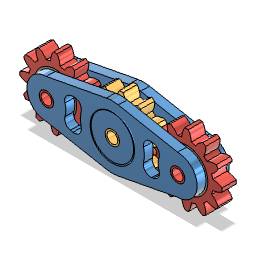
spur_gear_spinner (Autodesk Fusion 360 design; units mm, degrees)
Autodesk Fusion 360 part; units mm, degrees
sketch "Sketch1" plane through (0, 0, 0) normal (0, 0, 1) x (1, 0, 0)
  circle A0 centre (100, 50) radius 4
  circle A1 centre (174, 50) radius 4
  circle A2 centre (137.1972, 50) radius 12
  line L0 (100, 61) -> (133.8504, 67.3702)
  line L1 (140.5427, 67.3637) -> (174, 61)
  line L2 (100, 39) -> (133.8504, 32.6298)
  line L3 (140.5427, 32.6363) -> (174, 39)
  line L4 (113.559, 58.4638) -> (114.9878, 58.7327)
  line L5 (113.559, 41.5362) -> (114.9878, 41.2673)
  line L6 (159.425, 58.6826) -> (160.4563, 58.4864)
  line L7 (159.425, 41.3174) -> (160.4563, 41.5136)
  arc A3 (140.5427, 67.3637) -> (133.8504, 67.3702) centre (137.1794, 49.6807) ccw
  arc A4 (133.8504, 32.6298) -> (140.5427, 32.6363) centre (137.1794, 50.3193) ccw
  arc A5 (113.559, 58.4638) -> (110.4857, 53.3241) centre (114.2987, 54.5328) ccw
  arc A6 (119.6312, 53.9287) -> (114.9878, 58.7327) centre (115.7276, 54.8017) ccw
  arc A7 (100, 61) -> (100, 39) centre (100, 50) ccw
  arc A8 (110.4857, 46.6759) -> (110.4857, 53.3241) centre (100, 50) ccw
  arc A9 (119.6312, 53.9287) -> (119.6312, 46.0713) centre (137.1972, 50) ccw
  arc A10 (154.7721, 46.1112) -> (154.7721, 53.8888) centre (137.1972, 50) ccw
  arc A11 (163.5199, 53.3417) -> (163.5199, 46.6583) centre (174, 50) ccw
  arc A12 (174, 39) -> (174, 61) centre (174, 50) ccw
  arc A13 (110.4857, 46.6759) -> (113.559, 41.5362) centre (114.2987, 45.4672) ccw
  arc A14 (114.9878, 41.2673) -> (119.6312, 46.0713) centre (115.7276, 45.1983) ccw
  arc A15 (159.425, 58.6826) -> (154.7721, 53.8888) centre (158.6776, 54.753) ccw
  arc A16 (163.5199, 53.3417) -> (160.4563, 58.4864) centre (159.7089, 54.5569) ccw
  arc A17 (154.7721, 46.1112) -> (159.425, 41.3174) centre (158.6776, 45.247) ccw
  arc A18 (160.4563, 41.5136) -> (163.5199, 46.6583) centre (159.7089, 45.4431) ccw
  line L8 (300, 39) -> (266.1496, 32.6298)
  circle A19 centre (300, 50) radius 4
  arc A20 (266.1496, 67.3702) -> (259.4573, 67.3637) centre (262.8206, 49.6807) ccw
  arc A21 (240.575, 41.3174) -> (245.2279, 46.1112) centre (241.3224, 45.247) ccw
  line L9 (240.575, 58.6826) -> (239.5437, 58.4864)
  line L10 (259.4573, 32.6363) -> (226, 39)
  line L11 (300, 61) -> (266.1496, 67.3702)
  arc A22 (236.4801, 46.6583) -> (239.5437, 41.5136) centre (240.2911, 45.4431) ccw
  arc A23 (280.3688, 46.0713) -> (285.0122, 41.2673) centre (284.2724, 45.1983) ccw
  arc A24 (245.2279, 53.8888) -> (245.2279, 46.1112) centre (262.8028, 50) ccw
  arc A25 (286.441, 41.5362) -> (289.5143, 46.6759) centre (285.7013, 45.4672) ccw
  line L12 (286.441, 41.5362) -> (285.0122, 41.2673)
  arc A26 (239.5437, 58.4864) -> (236.4801, 53.3417) centre (240.2911, 54.5569) ccw
  arc A27 (289.5143, 53.3241) -> (289.5143, 46.6759) centre (300, 50) ccw
  arc A28 (245.2279, 53.8888) -> (240.575, 58.6826) centre (241.3224, 54.753) ccw
  arc A29 (285.0122, 58.7327) -> (280.3688, 53.9287) centre (284.2724, 54.8017) ccw
  line L13 (240.575, 41.3174) -> (239.5437, 41.5136)
  arc A30 (236.4801, 46.6583) -> (236.4801, 53.3417) centre (226, 50) ccw
  circle A31 centre (262.8028, 50) radius 12
  arc A32 (226, 61) -> (226, 39) centre (226, 50) ccw
  arc A33 (289.5143, 53.3241) -> (286.441, 58.4638) centre (285.7013, 54.5328) ccw
  arc A34 (259.4573, 32.6363) -> (266.1496, 32.6298) centre (262.8206, 50.3193) ccw
  arc A35 (300, 39) -> (300, 61) centre (300, 50) ccw
  circle A36 centre (226, 50) radius 4
  line L14 (259.4573, 67.3637) -> (226, 61)
  line L15 (286.441, 58.4638) -> (285.0122, 58.7327)
  arc A37 (280.3688, 46.0713) -> (280.3688, 53.9287) centre (262.8028, 50) ccw
  dimension "d1" = 22
  dimension "d2" = 8
  dimension "d3" = 22
  dimension "d4" = 8
  dimension "d5" = 74
  dimension "d6" = 36
  dimension "d7" = 24
  dimension "d8" = 5
  dimension "d9" = 5
  dimension "d11" = 5
  dimension "d12" = 5
  dimension "d13" = 18
  dimension "d14" = 18
  dimension "d15" = 4
  dimension "d16" = 4
  dimension "d17" = 4
  dimension "d18" = 4
  dimension "d19" = 4
  dimension "d20" = 4
  dimension "d21" = 4
  dimension "d22" = 4
  constraint concentric A0 A7
  constraint concentric A1 A11
  constraint concentric A2 A9
  constraint coincident L3.end A11
  constraint parallel L0 L4
  constraint parallel L2 L5
  constraint parallel L1 L6
  constraint parallel L3 L7
  constraint tangent L0 A3
  constraint tangent L1 A3
  constraint tangent L2 A4
  constraint tangent L3 A4
  constraint tangent A5 A7
  constraint tangent L4 A5
  constraint tangent L4 A6
  constraint tangent A6 A9
  constraint concentric A7 A8
  constraint concentric A9 A10
  constraint concentric A11 A12
  constraint tangent A8 A13
  constraint tangent L5 A13
  constraint tangent L5 A14
  constraint tangent A9 A14
  constraint tangent A10 A15
  constraint tangent L6 A15
  constraint tangent L6 A16
  constraint tangent A11 A16
  constraint tangent A10 A17
  constraint tangent L7 A17
  constraint tangent L7 A18
  constraint tangent A11 A18
  measures "d1" diameter of A7
  measures "d2" diameter of A0
  measures "d3" diameter of A11
  measures "d4" diameter of A1
  measures "d5" distance of A0.centre A1.centre
  measures "d6" diameter of A9
  measures "d7" diameter of A2
  measures "d8" distance of L0 L4
  measures "d9" distance of L2 L5
  measures "d11" distance of L1 L6
  measures "d12" distance of L3 L7
  measures "d13" radius of A3
  measures "d14" radius of A4
  measures "d15" radius of A5
  measures "d16" radius of A6
  measures "d17" radius of A13
  measures "d18" radius of A14
  measures "d19" radius of A15
  measures "d20" radius of A16
  measures "d21" radius of A17
  measures "d22" radius of A18
extrude "Extrude1" add sketch "Sketch1" along normal blind 5 contours L0 L1 L2 L3 A3 A4 A7 A12 makes body 1 in component "Top plate"
extrude "Extrude1'" add sketch "Sketch1" along normal blind 5 separate body contours L8 A20 L10 L11 A32 A34 A35 L14 makes body 2 in component "Bottom plate"
sketch "Sketch2" plane through (0, 0, 0) normal (0, 0, 1) x (1, 0, 0)
  circle A0 centre (98.0968, 130.2968) radius 12
  line L0 (97.0968, 150.2968) -> (99.0968, 150.2968)
  arc A1 (97.0968, 150.2968) -> (95.4218, 145.0564) centre (105.4171, 144.7495) ccw
  arc A2 (100.7718, 145.0564) -> (99.0968, 150.2968) centre (90.7765, 144.7495) ccw
  arc A3 (93.0336, 144.4165) -> (88.9628, 148.1173) centre (84.5309, 139.1531) ccw
  line L1 (87.2307, 147.1173) -> (88.9628, 148.1173)
  arc A4 (87.2307, 147.1173) -> (88.4004, 141.7415) centre (97.21, 146.4734) ccw
  arc A5 (86.6521, 139.9932) -> (81.2763, 141.1629) centre (81.9202, 131.1836) ccw
  line L2 (80.2763, 139.4308) -> (81.2763, 141.1629)
  arc A6 (80.2763, 139.4308) -> (83.9771, 135.36) centre (89.2405, 143.8627) ccw
  arc A7 (83.3372, 132.9718) -> (78.0968, 131.2968) centre (83.6441, 122.9765) ccw
  line L3 (78.0968, 129.2968) -> (78.0968, 131.2968)
  arc A8 (78.0968, 129.2968) -> (83.3372, 127.6218) centre (83.6441, 137.6171) ccw
  arc A9 (83.9771, 125.2337) -> (80.2763, 121.1629) centre (89.2405, 116.7309) ccw
  line L4 (81.2763, 119.4308) -> (80.2763, 121.1629)
  arc A10 (81.2763, 119.4308) -> (86.6521, 120.6004) centre (81.9202, 129.4101) ccw
  arc A11 (88.4004, 118.8522) -> (87.2307, 113.4763) centre (97.21, 114.1203) ccw
  line L5 (88.9628, 112.4763) -> (87.2307, 113.4763)
  arc A12 (88.9628, 112.4763) -> (93.0336, 116.1772) centre (84.5309, 121.4406) ccw
  arc A13 (95.4218, 115.5373) -> (97.0968, 110.2968) centre (105.4171, 115.8442) ccw
  line L6 (99.0968, 110.2968) -> (97.0968, 110.2968)
  arc A14 (99.0968, 110.2968) -> (100.7718, 115.5373) centre (90.7765, 115.8442) ccw
  arc A15 (103.1599, 116.1772) -> (107.2307, 112.4763) centre (111.6627, 121.4406) ccw
  line L7 (108.9628, 113.4763) -> (107.2307, 112.4763)
  arc A16 (108.9628, 113.4763) -> (107.7932, 118.8522) centre (98.9835, 114.1203) ccw
  arc A17 (109.5414, 120.6004) -> (114.9173, 119.4308) centre (114.2733, 129.4101) ccw
  line L8 (115.9173, 121.1629) -> (114.9173, 119.4308)
  arc A18 (115.9173, 121.1629) -> (112.2164, 125.2337) centre (106.953, 116.7309) ccw
  arc A19 (112.8563, 127.6218) -> (118.0968, 129.2968) centre (112.5494, 137.6171) ccw
  line L9 (118.0968, 131.2968) -> (118.0968, 129.2968)
  arc A20 (118.0968, 131.2968) -> (112.8563, 132.9718) centre (112.5494, 122.9765) ccw
  arc A21 (112.2164, 135.36) -> (115.9173, 139.4308) centre (106.953, 143.8627) ccw
  line L10 (114.9173, 141.1629) -> (115.9173, 139.4308)
  arc A22 (114.9173, 141.1629) -> (109.5414, 139.9932) centre (114.2733, 131.1836) ccw
  arc A23 (107.7932, 141.7415) -> (108.9628, 147.1173) centre (98.9835, 146.4734) ccw
  line L11 (107.2307, 148.1173) -> (108.9628, 147.1173)
  arc A24 (107.2307, 148.1173) -> (103.1599, 144.4165) centre (111.6627, 139.1531) ccw
  arc A25 (103.1599, 144.4165) -> (100.7718, 145.0564) centre (98.0968, 130.2968) ccw
  arc A26 (109.5414, 139.9932) -> (107.7932, 141.7415) centre (98.0968, 130.2968) ccw
  arc A27 (112.8563, 132.9718) -> (112.2164, 135.36) centre (98.0968, 130.2968) ccw
  arc A28 (112.2164, 125.2337) -> (112.8563, 127.6218) centre (98.0968, 130.2968) ccw
  arc A29 (107.7932, 118.8522) -> (109.5414, 120.6004) centre (98.0968, 130.2968) ccw
  arc A30 (100.7718, 115.5373) -> (103.1599, 116.1772) centre (98.0968, 130.2968) ccw
  arc A31 (93.0336, 116.1772) -> (95.4218, 115.5373) centre (98.0968, 130.2968) ccw
  arc A32 (86.6521, 120.6004) -> (88.4004, 118.8522) centre (98.0968, 130.2968) ccw
  arc A33 (83.3372, 127.6218) -> (83.9771, 125.2337) centre (98.0968, 130.2968) ccw
  arc A34 (83.9771, 135.36) -> (83.3372, 132.9718) centre (98.0968, 130.2968) ccw
  arc A35 (95.4218, 145.0564) -> (93.0336, 144.4165) centre (98.0968, 130.2968) ccw
  arc A36 (88.4004, 141.7415) -> (86.6521, 139.9932) centre (98.0968, 130.2968) ccw
  arc A37 (151.0372, 147.1173) -> (152.2068, 141.7415) centre (161.0165, 146.4734) ccw
  circle A38 centre (161.9032, 130.2968) radius 12
  arc A39 (164.5782, 145.0564) -> (162.9032, 150.2968) centre (154.5829, 144.7495) ccw
  arc A40 (173.3479, 139.9932) -> (171.5996, 141.7415) centre (161.9032, 130.2968) ccw
  arc A41 (176.0229, 135.36) -> (179.7237, 139.4308) centre (170.7595, 143.8627) ccw
  arc A42 (164.5782, 115.5373) -> (166.9664, 116.1772) centre (161.9032, 130.2968) ccw
  line L12 (172.7693, 147.1173) -> (171.0372, 148.1173)
  arc A43 (176.0229, 125.2337) -> (176.6628, 127.6218) centre (161.9032, 130.2968) ccw
  arc A44 (172.7693, 113.4763) -> (171.5996, 118.8522) centre (162.79, 114.1203) ccw
  arc A45 (171.5996, 118.8522) -> (173.3479, 120.6004) centre (161.9032, 130.2968) ccw
  line L13 (179.7237, 139.4308) -> (178.7237, 141.1629)
  arc A46 (171.5996, 141.7415) -> (172.7693, 147.1173) centre (162.79, 146.4734) ccw
  line L14 (181.9032, 129.2968) -> (181.9032, 131.2968)
  arc A47 (179.7237, 121.1629) -> (176.0229, 125.2337) centre (170.7595, 116.7309) ccw
  arc A48 (176.6628, 127.6218) -> (181.9032, 129.2968) centre (176.3559, 137.6171) ccw
  line L15 (178.7237, 119.4308) -> (179.7237, 121.1629)
  line L16 (144.0827, 121.1629) -> (145.0827, 119.4308)
  arc A49 (144.0827, 139.4308) -> (147.7836, 135.36) centre (153.047, 143.8627) ccw
  arc A50 (147.1437, 127.6218) -> (147.7836, 125.2337) centre (161.9032, 130.2968) ccw
  arc A51 (159.2282, 115.5373) -> (160.9032, 110.2968) centre (169.2235, 115.8442) ccw
  arc A52 (147.7836, 125.2337) -> (144.0827, 121.1629) centre (153.047, 116.7309) ccw
  line L17 (145.0827, 141.1629) -> (144.0827, 139.4308)
  arc A53 (147.7836, 135.36) -> (147.1437, 132.9718) centre (161.9032, 130.2968) ccw
  arc A54 (160.9032, 150.2968) -> (159.2282, 145.0564) centre (169.2235, 144.7495) ccw
  arc A55 (145.0827, 119.4308) -> (150.4586, 120.6004) centre (145.7267, 129.4101) ccw
  arc A56 (152.2068, 118.8522) -> (151.0372, 113.4763) centre (161.0165, 114.1203) ccw
  arc A57 (152.7693, 112.4763) -> (156.8401, 116.1772) centre (148.3373, 121.4406) ccw
  arc A58 (141.9032, 129.2968) -> (147.1437, 127.6218) centre (147.4506, 137.6171) ccw
  line L18 (141.9032, 131.2968) -> (141.9032, 129.2968)
  arc A59 (159.2282, 145.0564) -> (156.8401, 144.4165) centre (161.9032, 130.2968) ccw
  arc A60 (150.4586, 139.9932) -> (145.0827, 141.1629) centre (145.7267, 131.1836) ccw
  arc A61 (166.9664, 116.1772) -> (171.0372, 112.4763) centre (175.4691, 121.4406) ccw
  arc A62 (173.3479, 120.6004) -> (178.7237, 119.4308) centre (178.0798, 129.4101) ccw
  arc A63 (166.9664, 144.4165) -> (164.5782, 145.0564) centre (161.9032, 130.2968) ccw
  arc A64 (171.0372, 148.1173) -> (166.9664, 144.4165) centre (175.4691, 139.1531) ccw
  arc A65 (181.9032, 131.2968) -> (176.6628, 132.9718) centre (176.3559, 122.9765) ccw
  line L19 (152.7693, 148.1173) -> (151.0372, 147.1173)
  arc A66 (162.9032, 110.2968) -> (164.5782, 115.5373) centre (154.5829, 115.8442) ccw
  line L20 (171.0372, 112.4763) -> (172.7693, 113.4763)
  arc A67 (178.7237, 141.1629) -> (173.3479, 139.9932) centre (178.0798, 131.1836) ccw
  arc A68 (156.8401, 116.1772) -> (159.2282, 115.5373) centre (161.9032, 130.2968) ccw
  arc A69 (156.8401, 144.4165) -> (152.7693, 148.1173) centre (148.3373, 139.1531) ccw
  arc A70 (176.6628, 132.9718) -> (176.0229, 135.36) centre (161.9032, 130.2968) ccw
  line L21 (151.0372, 113.4763) -> (152.7693, 112.4763)
  arc A71 (147.1437, 132.9718) -> (141.9032, 131.2968) centre (147.4506, 122.9765) ccw
  arc A72 (152.2068, 141.7415) -> (150.4586, 139.9932) centre (161.9032, 130.2968) ccw
  arc A73 (150.4586, 120.6004) -> (152.2068, 118.8522) centre (161.9032, 130.2968) ccw
  line L22 (162.9032, 150.2968) -> (160.9032, 150.2968)
  line L23 (160.9032, 110.2968) -> (162.9032, 110.2968)
  dimension "d27" = 30
  dimension "d28" = 24
  dimension "d29" = 20
  dimension "d36" = 10
  dimension "d38" = 360
  constraint concentric A0 A35
  constraint horizontal L0
  constraint concentric A25 A35
  constraint concentric A26 A35
  constraint concentric A27 A35
  constraint concentric A28 A35
  constraint concentric A29 A35
  constraint concentric A30 A35
  constraint concentric A31 A35
  constraint concentric A32 A35
  constraint concentric A33 A35
  constraint concentric A34 A35
  constraint concentric A35 A36
  measures "d27" diameter of A35
  measures "d28" diameter of A0
  measures "d29" distance of A0.centre L0
  measures "d36" radius of A1
extrude "Extrude1''" add sketch "Sketch2" along normal blind 8 separate body contours L0 A1 A2 A3 L1 A4 A5 L2 A6 A7 L3 A8 A9 L4 A10 A11 L5 A12 A13 L6 A14 A15 L7 A16 A17 L8 A18 A19 L9 A20 A21 L10 A22 A23 L11 A24 A25 A26 A27 A28 A29 A30 A31 A32 A33 A34 A35 A36 makes body 3 in component "Spur Gear1/3"
extrude "Extrude1'''" add sketch "Sketch2" along normal blind 8 separate body contours A37 A39 A40 A41 A42 L12 A43 A44 A45 L13 A46 L14 A47 A48 L15 L16 A49 A50 A51 A52 L17 A53 A54 A55 A56 A57 A58 L18 A59 A60 A61 A62 A63 A64 A65 L19 A66 L20 A67 A68 A69 A70 L21 A71 A72 A73 L22 L23 makes body 4 in component "Spu Gear 2/3"
sketch "Sketch3" plane through (0, 0, 0) normal (0, 0, 1) x (1, 0, 0)
  circle A0 centre (243.1041, 130.2402) radius 4
  line L0 (242.1041, 150.2402) -> (244.1041, 150.2402)
  arc A1 (245.7791, 144.9998) -> (244.1041, 150.2402) centre (235.7838, 144.6929) ccw
  arc A2 (242.1041, 150.2402) -> (240.4291, 144.9998) centre (250.4244, 144.6929) ccw
  arc A3 (238.041, 144.3599) -> (233.9702, 148.0607) centre (229.5382, 139.0965) ccw
  arc A4 (232.2381, 147.0607) -> (233.4077, 141.6849) centre (242.2173, 146.4167) ccw
  line L1 (232.2381, 147.0607) -> (233.9702, 148.0607)
  arc A5 (231.6595, 139.9366) -> (226.2836, 141.1062) centre (226.9276, 131.127) ccw
  arc A6 (225.2836, 139.3742) -> (228.9845, 135.3034) centre (234.2479, 143.8061) ccw
  line L2 (225.2836, 139.3742) -> (226.2836, 141.1062)
  arc A7 (228.3446, 132.9152) -> (223.1041, 131.2402) centre (228.6514, 122.9199) ccw
  arc A8 (223.1041, 129.2402) -> (228.3446, 127.5652) centre (228.6514, 137.5605) ccw
  line L3 (223.1041, 129.2402) -> (223.1041, 131.2402)
  arc A9 (228.9845, 125.1771) -> (225.2836, 121.1062) centre (234.2479, 116.6743) ccw
  arc A10 (226.2836, 119.3742) -> (231.6595, 120.5438) centre (226.9276, 129.3534) ccw
  line L4 (226.2836, 119.3742) -> (225.2836, 121.1062)
  arc A11 (233.4077, 118.7956) -> (232.2381, 113.4197) centre (242.2173, 114.0637) ccw
  arc A12 (233.9702, 112.4197) -> (238.041, 116.1206) centre (229.5382, 121.384) ccw
  line L5 (233.9702, 112.4197) -> (232.2381, 113.4197)
  arc A13 (240.4291, 115.4807) -> (242.1041, 110.2402) centre (250.4244, 115.7875) ccw
  arc A14 (244.1041, 110.2402) -> (245.7791, 115.4807) centre (235.7838, 115.7875) ccw
  line L6 (244.1041, 110.2402) -> (242.1041, 110.2402)
  arc A15 (248.1673, 116.1206) -> (252.2381, 112.4197) centre (256.67, 121.384) ccw
  arc A16 (253.9702, 113.4197) -> (252.8005, 118.7956) centre (243.9909, 114.0637) ccw
  line L7 (253.9702, 113.4197) -> (252.2381, 112.4197)
  arc A17 (254.5488, 120.5438) -> (259.9246, 119.3742) centre (259.2807, 129.3534) ccw
  arc A18 (260.9246, 121.1062) -> (257.2238, 125.1771) centre (251.9604, 116.6743) ccw
  line L8 (260.9246, 121.1062) -> (259.9246, 119.3742)
  arc A19 (257.8637, 127.5652) -> (263.1041, 129.2402) centre (257.5568, 137.5605) ccw
  arc A20 (263.1041, 131.2402) -> (257.8637, 132.9152) centre (257.5568, 122.9199) ccw
  line L9 (263.1041, 131.2402) -> (263.1041, 129.2402)
  arc A21 (257.2238, 135.3034) -> (260.9246, 139.3742) centre (251.9604, 143.8061) ccw
  arc A22 (259.9246, 141.1062) -> (254.5488, 139.9366) centre (259.2807, 131.127) ccw
  line L10 (259.9246, 141.1062) -> (260.9246, 139.3742)
  arc A23 (252.8005, 141.6849) -> (253.9702, 147.0607) centre (243.9909, 146.4167) ccw
  arc A24 (252.2381, 148.0607) -> (248.1673, 144.3599) centre (256.67, 139.0965) ccw
  line L11 (252.2381, 148.0607) -> (253.9702, 147.0607)
  arc A25 (248.1673, 144.3599) -> (245.7791, 144.9998) centre (243.1041, 130.2402) ccw
  arc A26 (254.5488, 139.9366) -> (252.8005, 141.6849) centre (243.1041, 130.2402) ccw
  arc A27 (257.8637, 132.9152) -> (257.2238, 135.3034) centre (243.1041, 130.2402) ccw
  arc A28 (257.2238, 125.1771) -> (257.8637, 127.5652) centre (243.1041, 130.2402) ccw
  arc A29 (252.8005, 118.7956) -> (254.5488, 120.5438) centre (243.1041, 130.2402) ccw
  arc A30 (245.7791, 115.4807) -> (248.1673, 116.1206) centre (243.1041, 130.2402) ccw
  arc A31 (238.041, 116.1206) -> (240.4291, 115.4807) centre (243.1041, 130.2402) ccw
  arc A32 (231.6595, 120.5438) -> (233.4077, 118.7956) centre (243.1041, 130.2402) ccw
  arc A33 (228.3446, 127.5652) -> (228.9845, 125.1771) centre (243.1041, 130.2402) ccw
  arc A34 (228.9845, 135.3034) -> (228.3446, 132.9152) centre (243.1041, 130.2402) ccw
  arc A35 (240.4291, 144.9998) -> (238.041, 144.3599) centre (243.1041, 130.2402) ccw
  arc A36 (233.4077, 141.6849) -> (231.6595, 139.9366) centre (243.1041, 130.2402) ccw
  dimension "d43" = 30
  dimension "d44" = 8
  dimension "d45" = 20
  dimension "d51" = 10
  dimension "d53" = 360
  constraint concentric A0 A35
  constraint horizontal L0
  constraint concentric A25 A35
  constraint concentric A26 A35
  constraint concentric A27 A35
  constraint concentric A28 A35
  constraint concentric A29 A35
  constraint concentric A30 A35
  constraint concentric A31 A35
  constraint concentric A32 A35
  constraint concentric A33 A35
  constraint concentric A34 A35
  constraint concentric A35 A36
  measures "d43" diameter of A35
  measures "d44" diameter of A0
  measures "d45" distance of A0.centre L0
  measures "d51" radius of A1
extrude "Extrude1''''" add sketch "Sketch3" along normal blind 8 separate body makes body 5 in component "Spur Gear3/3"
sketch "Sketch4" plane through (0, 0, 0) normal (0, 0, 1) x (1, 0, 0)
  circle A0 centre (100, 200) radius 13
  circle A1 centre (100, 200) radius 4
  circle A2 centre (150, 200) radius 4
  circle A3 centre (150, 200) radius 13
  dimension "d56" = 26
  dimension "d57" = 8
  constraint concentric A0 A1
  measures "d56" diameter of A0
  measures "d57" diameter of A1
extrude "Extrude1'''''" add sketch "Sketch4" along normal blind 5 separate body contours A0 makes body 6 in component "major Base"
fillet "Fillet1" radius 0.5 1 edges at (87.8797, 195.299, 5) on bodies 6 in component "major Base"
fillet "Fillet2" radius 0.5 1 edges at (87.8797, 195.299, 0) on bodies 6 in component "major Base"
extrude "Extrude1''''''" add sketch "Sketch4" along normal blind 5 separate body contours A3 makes body 7 in component "pillor cap"
fillet "Fillet1'" radius 0.5 1 edges at (137.8797, 195.299, 5) on bodies 7 in component "pillor cap"
fillet "Fillet2'" radius 0.5 1 edges at (137.8797, 195.299, 0) on bodies 7 in component "pillor cap"
sketch "Sketch5" plane through (0, 0, 0) normal (0, 0, 1) x (1, 0, 0)
  circle A0 centre (200, 200) radius 4
  circle A1 centre (200, 200) radius 3
  circle A2 centre (220, 200) radius 3
  circle A3 centre (220, 200) radius 4
  circle A4 centre (240, 200) radius 3
  circle A5 centre (240, 200) radius 4
  circle A6 centre (100, 260) radius 12
  circle A7 centre (100, 260) radius 4
  circle A8 centre (150, 260) radius 4
  circle A9 centre (150, 260) radius 12
  dimension "d70" = 8
  dimension "d71" = 6
  dimension "d72" = 24
  dimension "d73" = 8
  constraint concentric A0 A1
  constraint concentric A6 A7
  measures "d70" diameter of A0
  measures "d71" diameter of A1
  measures "d72" diameter of A6
  measures "d73" diameter of A7
extrude "Extrude1'''''''" add sketch "Sketch5" along normal blind 18 separate body contours A0 makes body 8 in component "major Pillar"
extrude "Extrude1''''''''" add sketch "Sketch5" along normal blind 18 separate body contours A3 makes body 9 in component "minor pillar 1/2"
extrude "Extrude1'''''''''" add sketch "Sketch5" along normal blind 18 separate body contours A5 makes body 10 in component "minor pillar 2/2"
extrude "Extrude1''''''''''" add sketch "Sketch5" along normal blind 8 separate body contours A6 makes body 11 in component "Component"
extrude "Extrude1'''''''''''" add sketch "Sketch5" along normal blind 8 separate body contours A9 makes body 12 in component "Component'"
component "Top plate" placed x (1, 0, 0) y (0, 1, 0) z (0, 0, 1) at (0, 0, 0)
component "Bottom plate" placed x (1, 0, 0) y (0, 1, 0) z (0, 0, 1) at (-126, 0, -13)
component "Spur Gear1/3" placed x (1, 0, 0) y (0, 1, 0) z (0, 0, 1) at (1.9032, -80.2968, -8)
component "Spu Gear 2/3" placed x (1, 0, 0) y (0, 1, 0) z (0, 0, 1) at (12.0968, -80.2968, -8)
component "Spur Gear3/3" placed x (1, 0, 0) y (0, 1, 0) z (0, 0, 1) at (-105.9248, -80.5595, -8)
component "major Base" placed x (1, 0, 0) y (0, 1, 0) z (0, 0, 1) at (37.1794, -150.3193, -13)
component "pillor cap" placed x (1, 0, 0) y (0, 1, 0) z (0, 0, 1) at (-12.8206, -150.3193, 0)
component "major Pillar" placed x (1, 0, 0) y (0, 1, 0) z (0, 0, 1) at (-62.8206, -150.3193, -13)
component "minor pillar 1/2" placed x (1, 0, 0) y (0, 1, 0) z (0, 0, 1) at (-120, -150, -13)
component "minor pillar 2/2" placed x (1, 0, 0) y (0, 1, 0) z (0, 0, 1) at (-66, -150, -13)
component "Component" placed x (1, 0, 0) y (0, 1, 0) z (0, 0, 1) at (0, -210, -8)
component "Component'" placed x (1, 0, 0) y (0, 1, 0) z (0, 0, 1) at (24, -210, -8)
